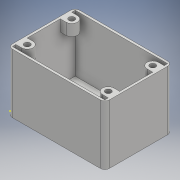
# Autodesk Inventor part: CASE ESP32 CAM
Saved by Autodesk Inventor 2018 (Build 220112000, 112)
## iProperties
Created: 2022-03-14
Part Number: CASE ESP32 CAM
Material: Genérico
Document SubType Name: Modeling
Designer: ADM
Density: 1 g/cm^3
Appearance: Padrão
Author: ADM
Autodesk Inventor part; units mm, degrees
ref_plane "YZ Plane" through (0, 0, 0) normal (1, 0, 0) x (0, 1, 0)
ref_plane "XZ Plane" through (0, 0, 0) normal (0, 1, 0) x (-1, 0, 0)
ref_plane "XY Plane" through (0, 0, 0) normal (0, 0, 1) x (1, 0, 0)
sketch "Esboço1" plane through (0, 0, 0) normal (0, 1, 0) x (-1, 0, 0)
  point P0 (0, 0)
sketch "Esboço2" plane through (0, 0, 0) normal (0, 0, 1) x (1, 0, 0)
  line L0 (0, 0) -> (40.5, 0)
  line L1 (40.5, 0) -> (40.5, 27.5)
  line L2 (40.5, 27.5) -> (0, 27.5)
  line L3 (0, 27.5) -> (0, 0)
  line L4 (40.5, 27.5) -> (32.5, 27.5)
  line L5 (28.5, 13.75) -> (28.5, 17.75)
  line L6 (28.5, 13.75) -> (28.5, 9.75)
  line L7 (36.5, 13.75) -> (36.5, 17.75)
  line L8 (36.5, 13.75) -> (36.5, 9.75)
  line L9 (36.5, 17.75) -> (28.5, 17.75)
  line L10 (36.5, 9.75) -> (28.5, 9.75)
  dimension "d3" = 40.5
  dimension "d4" = 27.5
  dimension "d5" = 8
  dimension "d9" = 4
  dimension "d10" = 4
  constraints: 22 end point, 4 vertical, 3 perpendicular, 1 horizontal, 1 point on line
  measures "d3" distance of L0.start L0.end
  measures "d4" distance of L0.end L1.end
  measures "d5" distance of L1.end L4.end
  measures "d9" distance of L5.start L5.end
  measures "d10" distance of L5.start L6.end
extrude "Extrusão1" add sketch "Esboço2" along normal blind 25
shell "Casca1" thickness 1 outward yes removed faces 7 at (9.5, 13.75, 25) at (33.8333, 9.75, 8.3333) at (28.5, 11.0833, 8.3333) at (28.5, 15.0833, 8.3333) at (31.1667, 17.75, 8.3333) at (36.5, 12.4167, 8.3333) at (36.5, 16.4167, 8.3333)
fillet "Arredondamento1" radius 2 4 edges at (-1, -1, 12) (41.5, -1, 12) (41.5, 28.5, 12) (-1, 28.5, 12)
sketch "Esboço3" plane through (0, 0, -1) normal (0, 0, -1) x (-1, 0, 0)
  line L0 (-25.972, 15.6624) -> (-1.7685, 15.6624) construction
  line L1 (-1.7685, 15.6624) -> (-1.7685, 10.822) construction
  line L2 (-1.7685, 10.822) -> (-25.972, 10.822) construction
  line L3 (-25.972, 10.822) -> (-25.972, 15.6624) construction
  line L4 (-25.6632, 12.5502) -> (-25.6632, 15.5982)
  line L5 (-25.6632, 15.5982) -> (-23.7564, 15.5982)
  line L6 (-23.7564, 15.5982) -> (-23.7564, 15.2376)
  line L7 (-23.7564, 15.2376) -> (-25.2581, 15.2376)
  line L8 (-25.2581, 15.2376) -> (-25.2581, 14.4027)
  line L9 (-25.2581, 14.4027) -> (-23.8576, 14.4027)
  line L10 (-23.8576, 14.4027) -> (-23.8576, 14.0421)
  line L11 (-23.8576, 14.0421) -> (-25.2581, 14.0421)
  line L12 (-25.2581, 14.0421) -> (-25.2581, 12.9108)
  line L13 (-25.2581, 12.9108) -> (-23.7564, 12.9108)
  line L14 (-23.7564, 12.9108) -> (-23.7564, 12.5502)
  line L15 (-23.7564, 12.5502) -> (-25.6632, 12.5502)
  spline S0 degree 2 poles (-22.4621, 12.4959) (-22.7931, 12.4959) (-23.2574, 12.6342) (-23.4624, 12.733) knots 0 0 0 1 2 2 2
  line L16 (-23.4624, 12.733) -> (-23.4624, 13.2418)
  line L17 (-23.4624, 13.2418) -> (-23.4328, 13.2418)
  spline S1 degree 2 poles (-23.4328, 13.2418) (-23.2327, 13.0541) (-22.7264, 12.8466) (-22.4917, 12.8466) knots 0 0 0 1 2 2 2
  spline S2 degree 2 poles (-22.4917, 12.8466) (-22.1558, 12.8466) (-21.8125, 13.1257) (-21.8125, 13.3554) knots 0 0 0 1 2 2 2
  spline S3 degree 2 poles (-21.8125, 13.3554) (-21.8125, 13.5382) (-21.9928, 13.7655) (-22.1879, 13.8223) knots 0 0 0 1 2 2 2
  spline S4 degree 2 poles (-22.1879, 13.8223) (-22.3287, 13.8618) (-22.5633, 13.9161) (-22.7387, 13.9606) knots 0 0 0 1 2 2 2
  spline S5 degree 2 poles (-22.7387, 13.9606) (-22.8968, 14.0026) (-23.1463, 14.1285) (-23.2426, 14.2298) knots 0 0 0 1 2 2 2
  spline S6 degree 2 poles (-23.2426, 14.2298) (-23.3365, 14.3311) (-23.4402, 14.6028) (-23.4402, 14.7806) knots 0 0 0 1 2 2 2
  spline S7 degree 2 poles (-23.4402, 14.7806) (-23.4402, 15.1511) (-22.8622, 15.6525) (-22.4151, 15.6525) knots 0 0 0 1 2 2 2
  spline S8 degree 2 poles (-22.4151, 15.6525) (-22.1583, 15.6525) (-21.7038, 15.5513) (-21.5087, 15.4549) knots 0 0 0 1 2 2 2
  line L18 (-21.5087, 15.4549) -> (-21.5087, 14.9708)
  line L19 (-21.5087, 14.9708) -> (-21.5383, 14.9708)
  spline S9 degree 2 poles (-21.5383, 14.9708) (-21.684, 15.1042) (-22.1385, 15.3018) (-22.388, 15.3018) knots 0 0 0 1 2 2 2
  spline S10 degree 2 poles (-22.388, 15.3018) (-22.6696, 15.3018) (-23.0178, 15.0375) (-23.0178, 14.8226) knots 0 0 0 1 2 2 2
  spline S11 degree 2 poles (-23.0178, 14.8226) (-23.0178, 14.63) (-22.8128, 14.4002) (-22.6202, 14.3484) knots 0 0 0 1 2 2 2
  spline S12 degree 2 poles (-22.6202, 14.3484) (-22.4917, 14.3138) (-22.1187, 14.2249) (-21.9952, 14.1878) knots 0 0 0 1 2 2 2
  spline S13 degree 2 poles (-21.9952, 14.1878) (-21.6816, 14.0915) (-21.3901, 13.7037) (-21.3901, 13.4196) knots 0 0 0 1 2 2 2
  spline S14 degree 2 poles (-21.3901, 13.4196) (-21.3901, 13.2393) (-21.5358, 12.8935) (-21.6667, 12.7725) knots 0 0 0 1 2 2 2
  spline S15 degree 2 poles (-21.6667, 12.7725) (-21.8125, 12.6391) (-22.183, 12.4959) (-22.4621, 12.4959) knots 0 0 0 1 2 2 2
  spline S16 degree 2 poles (-19.051, 14.6794) (-19.051, 14.4818) (-19.1918, 14.1261) (-19.3177, 14.0026) knots 0 0 0 1 2 2 2
  spline S17 degree 2 poles (-19.3177, 14.0026) (-19.4758, 13.847) (-19.9031, 13.6864) (-20.2292, 13.6864) knots 0 0 0 1 2 2 2
  line L20 (-20.2292, 13.6864) -> (-20.5725, 13.6864)
  line L21 (-20.5725, 13.6864) -> (-20.5725, 12.5502)
  line L22 (-20.5725, 12.5502) -> (-20.9776, 12.5502)
  line L23 (-20.9776, 12.5502) -> (-20.9776, 15.5982)
  line L24 (-20.9776, 15.5982) -> (-20.2119, 15.5982)
  spline S18 degree 2 poles (-20.2119, 15.5982) (-19.9402, 15.5982) (-19.5598, 15.5093) (-19.4141, 15.408) knots 0 0 0 1 2 2 2
  spline S19 degree 2 poles (-19.4141, 15.408) (-19.2436, 15.2919) (-19.051, 14.9338) (-19.051, 14.6794) knots 0 0 0 1 2 2 2
  spline S20 degree 2 poles (-19.4734, 14.667) (-19.4734, 14.8251) (-19.582, 15.0573) (-19.6932, 15.1314) knots 0 0 0 1 2 2 2
  spline S21 degree 2 poles (-19.6932, 15.1314) (-19.7895, 15.1956) (-20.0464, 15.2475) (-20.2366, 15.2475) knots 0 0 0 1 2 2 2
  line L25 (-20.2366, 15.2475) -> (-20.5725, 15.2475)
  line L26 (-20.5725, 15.2475) -> (-20.5725, 14.0322)
  line L27 (-20.5725, 14.0322) -> (-20.2959, 14.0322)
  spline S22 degree 2 poles (-20.2959, 14.0322) (-20.0489, 14.0322) (-19.7451, 14.1113) (-19.6463, 14.215) knots 0 0 0 1 2 2 2
  spline S23 degree 2 poles (-19.6463, 14.215) (-19.5549, 14.3064) (-19.4734, 14.5213) (-19.4734, 14.667) knots 0 0 0 1 2 2 2
  spline S24 degree 2 poles (-17.9296, 15.3092) (-18.0408, 15.3092) (-18.2606, 15.2549) (-18.3668, 15.2129) knots 0 0 0 1 2 2 2
  spline S25 degree 2 poles (-18.3668, 15.2129) (-18.4656, 15.1709) (-18.6113, 15.082) (-18.6681, 15.0424) knots 0 0 0 1 2 2 2
  line L28 (-18.6681, 15.0424) -> (-18.6928, 15.0424)
  line L29 (-18.6928, 15.0424) -> (-18.6928, 15.4747)
  spline S26 degree 2 poles (-18.6928, 15.4747) (-18.5595, 15.5463) (-18.1025, 15.6624) (-17.8975, 15.6624) knots 0 0 0 1 2 2 2
  spline S27 degree 2 poles (-17.8975, 15.6624) (-17.69, 15.6624) (-17.3813, 15.5784) (-17.2553, 15.4895) knots 0 0 0 1 2 2 2
  spline S28 degree 2 poles (-17.2553, 15.4895) (-17.1219, 15.3932) (-16.9836, 15.1141) (-16.9836, 14.9264) knots 0 0 0 1 2 2 2
  spline S29 degree 2 poles (-16.9836, 14.9264) (-16.9836, 14.6744) (-17.3146, 14.294) (-17.5467, 14.2446) knots 0 0 0 1 2 2 2
  line L30 (-17.5467, 14.2446) -> (-17.5467, 14.215)
  spline S30 degree 2 poles (-17.5467, 14.215) (-17.4504, 14.1952) (-17.2306, 14.1063) (-17.1367, 14.0174) knots 0 0 0 1 2 2 2
  spline S31 degree 2 poles (-17.1367, 14.0174) (-17.0429, 13.9309) (-16.9243, 13.6543) (-16.9243, 13.4542) knots 0 0 0 1 2 2 2
  spline S32 degree 2 poles (-16.9243, 13.4542) (-16.9243, 13.2492) (-17.0651, 12.9009) (-17.1935, 12.7676) knots 0 0 0 1 2 2 2
  spline S33 degree 2 poles (-17.1935, 12.7676) (-17.3269, 12.6292) (-17.7048, 12.486) (-17.9444, 12.486) knots 0 0 0 1 2 2 2
  spline S34 degree 2 poles (-17.9444, 12.486) (-18.1741, 12.486) (-18.6237, 12.5971) (-18.7768, 12.6737) knots 0 0 0 1 2 2 2
  line L31 (-18.7768, 12.6737) -> (-18.7768, 13.106)
  line L32 (-18.7768, 13.106) -> (-18.7472, 13.106)
  spline S35 degree 2 poles (-18.7472, 13.106) (-18.6187, 13.0121) (-18.184, 12.8392) (-17.9691, 12.8392) knots 0 0 0 1 2 2 2
  spline S36 degree 2 poles (-17.9691, 12.8392) (-17.8431, 12.8392) (-17.5912, 12.9182) (-17.5072, 13.0096) knots 0 0 0 1 2 2 2
  spline S37 degree 2 poles (-17.5072, 13.0096) (-17.4257, 13.101) (-17.3393, 13.3184) (-17.3393, 13.4839) knots 0 0 0 1 2 2 2
  spline S38 degree 2 poles (-17.3393, 13.4839) (-17.3393, 13.6494) (-17.4356, 13.8643) (-17.522, 13.926) knots 0 0 0 1 2 2 2
  spline S39 degree 2 poles (-17.522, 13.926) (-17.6085, 13.9878) (-17.8431, 14.0347) (-17.9815, 14.0347) knots 0 0 0 1 2 2 2
  line L33 (-17.9815, 14.0347) -> (-18.1544, 14.0347)
  line L34 (-18.1544, 14.0347) -> (-18.1544, 14.3731)
  line L35 (-18.1544, 14.3731) -> (-18.0185, 14.3731)
  spline S40 degree 2 poles (-18.0185, 14.3731) (-17.7443, 14.3731) (-17.3985, 14.6349) (-17.3985, 14.8844) knots 0 0 0 1 2 2 2
  spline S41 degree 2 poles (-17.3985, 14.8844) (-17.3985, 15.0005) (-17.4875, 15.166) (-17.5591, 15.2154) knots 0 0 0 1 2 2 2
  spline S42 degree 2 poles (-17.5591, 15.2154) (-17.6357, 15.2672) (-17.8234, 15.3092) (-17.9296, 15.3092) knots 0 0 0 1 2 2 2
  line L36 (-14.5852, 12.5502) -> (-16.4649, 12.5502)
  line L37 (-16.4649, 12.5502) -> (-16.4649, 12.9825)
  spline S43 degree 2 poles (-16.4649, 12.9825) (-16.2623, 13.1726) (-15.9017, 13.5259) (-15.7288, 13.7161) knots 0 0 0 1 2 2 2
  spline S44 degree 2 poles (-15.7288, 13.7161) (-15.3805, 14.0989) (-15.1261, 14.5583) (-15.1261, 14.8029) knots 0 0 0 1 2 2 2
  spline S45 degree 2 poles (-15.1261, 14.8029) (-15.1261, 14.9313) (-15.2052, 15.124) (-15.2768, 15.1857) knots 0 0 0 1 2 2 2
  spline S46 degree 2 poles (-15.2768, 15.1857) (-15.3484, 15.2475) (-15.5362, 15.3092) (-15.6498, 15.3092) knots 0 0 0 1 2 2 2
  spline S47 degree 2 poles (-15.6498, 15.3092) (-15.7585, 15.3092) (-15.9808, 15.2549) (-16.082, 15.2129) knots 0 0 0 1 2 2 2
  spline S48 degree 2 poles (-16.082, 15.2129) (-16.1685, 15.1783) (-16.329, 15.0795) (-16.3784, 15.0449) knots 0 0 0 1 2 2 2
  line L38 (-16.3784, 15.0449) -> (-16.4007, 15.0449)
  line L39 (-16.4007, 15.0449) -> (-16.4007, 15.4796)
  spline S49 degree 2 poles (-16.4007, 15.4796) (-16.2747, 15.5414) (-15.8227, 15.6624) (-15.6201, 15.6624) knots 0 0 0 1 2 2 2
  spline S50 degree 2 poles (-15.6201, 15.6624) (-15.1928, 15.6624) (-14.7112, 15.2104) (-14.7112, 14.8251) knots 0 0 0 1 2 2 2
  spline S51 degree 2 poles (-14.7112, 14.8251) (-14.7112, 14.6448) (-14.7951, 14.3434) (-14.8692, 14.215) knots 0 0 0 1 2 2 2
  spline S52 degree 2 poles (-14.8692, 14.215) (-14.9433, 14.0816) (-15.1582, 13.8198) (-15.2768, 13.6938) knots 0 0 0 1 2 2 2
  spline S53 degree 2 poles (-15.2768, 13.6938) (-15.4695, 13.4839) (-15.9412, 13.0343) (-16.082, 12.9034) knots 0 0 0 1 2 2 2
  line L40 (-16.082, 12.9034) -> (-14.5852, 12.9034)
  line L41 (-14.5852, 12.9034) -> (-14.5852, 12.5502)
  spline S54 degree 2 poles (-11.5915, 12.4959) (-11.8879, 12.4959) (-12.3894, 12.6959) (-12.5721, 12.896) knots 0 0 0 1 2 2 2
  spline S55 degree 2 poles (-12.5721, 12.896) (-12.7549, 13.0936) (-12.955, 13.6864) (-12.955, 14.0717) knots 0 0 0 1 2 2 2
  spline S56 degree 2 poles (-12.955, 14.0717) (-12.955, 14.4546) (-12.7599, 15.0227) (-12.5746, 15.2326) knots 0 0 0 1 2 2 2
  spline S57 degree 2 poles (-12.5746, 15.2326) (-12.3918, 15.4377) (-11.8929, 15.6525) (-11.5841, 15.6525) knots 0 0 0 1 2 2 2
  spline S58 degree 2 poles (-11.5841, 15.6525) (-11.431, 15.6525) (-11.1618, 15.6081) (-11.0481, 15.5735) knots 0 0 0 1 2 2 2
  spline S59 degree 2 poles (-11.0481, 15.5735) (-10.9493, 15.5414) (-10.7443, 15.45) (-10.6431, 15.3957) knots 0 0 0 1 2 2 2
  line L42 (-10.6431, 15.3957) -> (-10.6431, 14.9066)
  line L43 (-10.6431, 14.9066) -> (-10.6752, 14.9066)
  spline S60 degree 2 poles (-10.6752, 14.9066) (-10.7295, 14.956) (-10.8975, 15.0943) (-11.0185, 15.161) knots 0 0 0 1 2 2 2
  spline S61 degree 2 poles (-11.0185, 15.161) (-11.1346, 15.2252) (-11.4088, 15.3067) (-11.5866, 15.3067) knots 0 0 0 1 2 2 2
  spline S62 degree 2 poles (-11.5866, 15.3067) (-11.7817, 15.3067) (-12.13, 15.1462) (-12.2609, 14.993) knots 0 0 0 1 2 2 2
  spline S63 degree 2 poles (-12.2609, 14.993) (-12.3894, 14.8374) (-12.5326, 14.3657) (-12.5326, 14.0717) knots 0 0 0 1 2 2 2
  spline S64 degree 2 poles (-12.5326, 14.0717) (-12.5326, 13.758) (-12.3819, 13.306) (-12.251, 13.1504) knots 0 0 0 1 2 2 2
  spline S65 degree 2 poles (-12.251, 13.1504) (-12.1226, 12.9997) (-11.7793, 12.8466) (-11.5866, 12.8466) knots 0 0 0 1 2 2 2
  spline S66 degree 2 poles (-11.5866, 12.8466) (-11.4112, 12.8466) (-11.1124, 12.9331) (-10.9963, 12.9973) knots 0 0 0 1 2 2 2
  spline S67 degree 2 poles (-10.9963, 12.9973) (-10.8851, 13.0615) (-10.7196, 13.1949) (-10.6727, 13.2418) knots 0 0 0 1 2 2 2
  line L44 (-10.6727, 13.2418) -> (-10.6431, 13.2418)
  line L45 (-10.6431, 13.2418) -> (-10.6431, 12.7577)
  spline S68 degree 2 poles (-10.6431, 12.7577) (-10.7443, 12.7108) (-10.9222, 12.6243) (-11.0481, 12.5848) knots 0 0 0 1 2 2 2
  spline S69 degree 2 poles (-11.0481, 12.5848) (-11.1815, 12.5403) (-11.4088, 12.4959) (-11.5915, 12.4959) knots 0 0 0 1 2 2 2
  line L46 (-10.5937, 12.5502) -> (-9.5661, 15.5982)
  line L47 (-9.5661, 15.5982) -> (-9.0672, 15.5982)
  line L48 (-9.0672, 15.5982) -> (-8.0397, 12.5502)
  line L49 (-8.0397, 12.5502) -> (-8.467, 12.5502)
  line L50 (-8.467, 12.5502) -> (-8.7436, 13.4024)
  line L51 (-8.7436, 13.4024) -> (-9.907, 13.4024)
  line L52 (-9.907, 13.4024) -> (-10.1836, 12.5502)
  line L53 (-10.1836, 12.5502) -> (-10.5937, 12.5502)
  line L54 (-8.8548, 13.7482) -> (-9.3265, 15.1832)
  line L55 (-9.3265, 15.1832) -> (-9.7958, 13.7482)
  line L56 (-9.7958, 13.7482) -> (-8.8548, 13.7482)
  line L57 (-5.1374, 12.5502) -> (-5.5425, 12.5502)
  line L58 (-5.5425, 12.5502) -> (-5.5425, 15.1758)
  line L59 (-5.5425, 15.1758) -> (-6.3378, 13.39)
  line L60 (-6.3378, 13.39) -> (-6.5848, 13.39)
  line L61 (-6.5848, 13.39) -> (-7.3728, 15.1758)
  line L62 (-7.3728, 15.1758) -> (-7.3728, 12.5502)
  line L63 (-7.3728, 12.5502) -> (-7.7507, 12.5502)
  line L64 (-7.7507, 12.5502) -> (-7.7507, 15.5982)
  line L65 (-7.7507, 15.5982) -> (-7.1974, 15.5982)
  line L66 (-7.1974, 15.5982) -> (-6.4366, 13.9013)
  line L67 (-6.4366, 13.9013) -> (-5.7005, 15.5982)
  line L68 (-5.7005, 15.5982) -> (-5.1374, 15.5982)
  line L69 (-5.1374, 15.5982) -> (-5.1374, 12.5502)
  point P0 (0, 0)
  constraints: 2 other
emboss "Relevo1" sketch "Esboço3" operation add depth 0.5 direction (0, 0, 1)
sketch "Esboço4" plane through (0, 0, -1) normal (0, 0, -1) x (-1, 0, 0)
  point P0 (0, 0)
sketch "Esboço5" plane through (-1, 1, -1) normal (-1, 0, 0) x (0, 0, 1)
  point P0 (1, -1)
ref_plane "Plano de trabalho1" through (40.5, 0, 0) normal (-1, 0, 0) x (0, 0, 1)
sketch "Esboço6" plane through (40.5, 0, 0) normal (-1, 0, 0) x (0, 0, 1)
  line L0 (25, 28.5) -> (-1, 28.5) projected
  line L1 (25, 28.5) -> (25, 23.5)
  line L2 (25, 27.5) -> (25, 0) projected
  line L3 (20, 23.5) -> (20, 21)
  line L4 (20, 23.5) -> (20, 26)
  line L5 (20, 26) -> (25, 26)
  line L6 (20, 21) -> (25, 21)
  line L7 (25, -1) -> (25, 4)
  line L8 (20, 4) -> (20, 6.5)
  line L9 (20, 4) -> (20, 1.5)
  line L10 (20, 1.5) -> (25, 1.5)
  line L11 (20, 6.5) -> (25, 6.5)
  point P0 (0, 0)
  dimension "d20" = 5
  dimension "d21" = 5
  dimension "d22" = 2.5
  dimension "d23" = 2.5
  dimension "d24" = 5
  dimension "d25" = 5
  dimension "d26" = 2.5
  dimension "d27" = 2.5
  constraints: 20 end point, 5 point on line, 3 perpendicular, 3 vertical, 1 midpoint
  measures "d20" distance of L0.start L1.end
  measures "d21" distance of L1.end L3.start
  measures "d22" distance of L3.start L3.end
  measures "d23" distance of L3.start L4.end
  measures "d24" distance of L7.start L7.end
  measures "d25" distance of L7.end L8.start
  measures "d26" distance of L8.start L8.end
  measures "d27" distance of L8.start L9.end
extrude "Extrusão2" add sketch "Esboço6" along normal blind 5
fillet "Arredondamento2" radius 2.5 4 edges at (35.5, 26, 22.5) (35.5, 21, 22.5) (35.5, 6.5, 22.5) (35.5, 1.5, 22.5)
ref_plane "Plano de trabalho2" through (0, 0, 0) normal (1, 0, 0) x (0, 0, -1)
sketch "Esboço7" plane through (0, 0, 0) normal (1, 0, 0) x (0, 0, -1)
  line L0 (-25, 28.5) -> (-25, 23.5)
  line L1 (-20, 21) -> (-20, 26) projected
  line L2 (-20, 23.5) -> (-20, 26)
  line L3 (-20, 23.5) -> (-20, 21)
  line L4 (-20, 26) -> (-25, 26)
  line L5 (-20, 21) -> (-25, 21)
  line L6 (-25, 0) -> (-25, 27.5) projected
  line L7 (-25, -1) -> (-25, 4)
  line L8 (-25, 1.5) -> (-25, 6.5) projected
  line L9 (-20, 4) -> (-20, 6.5)
  line L10 (-20, 6.5) -> (-20, 1.5)
  line L11 (-25, 1.5) -> (-20, 1.5) projected
  line L12 (-20, 1.5) -> (-25, 1.5)
  line L13 (-20, 1.5) -> (-20, 6.5) projected
  line L14 (-20, 6.5) -> (-25, 6.5) projected
  line L15 (-20, 6.5) -> (-25, 6.5)
  point P0 (0, 0)
  dimension "d32" = 5
  dimension "d33" = 5
  dimension "d34" = 2.5
  dimension "d35" = 2.5
  dimension "d36" = 5
  dimension "d37" = 5
  dimension "d38" = 2.5
  dimension "d39" = 5
  constraints: 20 end point, 2 midpoint, 2 point on line, 1 collinear, 1 horizontal, 1 perpendicular, 1 vertical
  measures "d32" distance of L0.start L0.end
  measures "d33" distance of L0.end L2.start
  measures "d34" distance of L2.start L1.end
  measures "d35" distance of L2.start L1.start
  measures "d36" distance of L7.start L7.end
  measures "d37" distance of L7.end L9.start
  measures "d38" distance of L9.start L9.end
  measures "d39" distance of L9.end L10.end
extrude "Extrusão3" add sketch "Esboço7" along normal blind 5
fillet "Arredondamento3" radius 2.5 4 edges at (5, 26, 22.5) (5, 21, 22.5) (5, 6.5, 22.5) (5, 1.5, 22.5)
ref_plane "Plano de trabalho3" through (0, 0, 25) normal (0, 0, 1) x (1, 0, 0)
sketch "Esboço8" plane through (0, 0, 25) normal (0, 0, 1) x (1, 0, 0)
  line L0 (40.5, 21) -> (40.5, 26) projected
  line L1 (40.5, 23.5) -> (38, 23.5)
  line L2 (40.5, 1.5) -> (40.5, 6.5) projected
  line L3 (40.5, 4) -> (38, 4)
  line L4 (0, 6.5) -> (0, 1.5) projected
  line L5 (0, 4) -> (2.5, 4)
  line L6 (0, 23.5) -> (2.5, 23.5)
  circle A0 centre (38, 23.5) radius 1.25
  circle A1 centre (38, 4) radius 1.25
  circle A2 centre (2.5, 4) radius 1.25
  circle A3 centre (2.5, 23.5) radius 1.25
  point P0 (0, 0)
  dimension "d44" = 2.5
  dimension "d45" = 2.5
  dimension "d46" = 2.5
  dimension "d47" = 2.5
  dimension "d49" = 2.5
  dimension "d50" = 2.5
  dimension "d51" = 2.5
  dimension "d52" = 2.5
  constraints: 8 end point, 4 centre point, 4 coincident, 4 horizontal, 3 midpoint
  measures "d44" distance of L1.start L1.end
  measures "d45" distance of L3.start L3.end
  measures "d46" distance of L5.start L5.end
  measures "d47" distance of L6.start L6.end
  measures "d49" diameter of A0
  measures "d50" diameter of A1
  measures "d51" diameter of A2
  measures "d52" diameter of A3
hole "Furo1" at (38, 23.5, 25) at (38, 4, 25) at (2.5, 4, 25) at (2.5, 23.5, 25) direction (0, 0, -1) diameter 2.5 depth 3.5 tip angle 118
